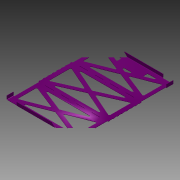
# Autodesk Inventor part: Base
Saved by Autodesk Inventor 2014 (Build 180170000, 170)
## iProperties
Created: 2014-01-11
Part Number: Base
Material: Aluminum 6061
Document SubType Name: Sheet Metal
Designer: Alex
Density: 2.71 g/cm^3
Sheet Metal Rule: Default
Appearance: Smooth - Purple
Mass: 1183.5 g
Surface Area: 4063.5 cm^2
Volume: 436.714 cm^3
Author: Alex
Autodesk Inventor part; units mm, degrees
ref_plane "YZ Plane" through (0, 0, 0) normal (1, 0, 0) x (0, 1, 0)
ref_plane "XZ Plane" through (0, 0, 0) normal (0, 1, 0) x (-1, 0, 0)
ref_plane "XY Plane" through (0, 0, 0) normal (0, 0, 1) x (1, 0, 0)
sketch "Sketch1" plane through (0, 0, 0) normal (0, 1, 0) x (-1, 0, 0)
  line L0 (-666.279, 180.2846) -> (-168.6422, 180.2846)
  line L1 (-168.6422, 180.2846) -> (-168.6422, -512.1194)
  line L2 (-168.6422, -512.1194) -> (-666.279, -512.1194)
  line L3 (-666.279, -512.1194) -> (-666.279, 180.2846)
  line L4 (-666.279, 180.2846) -> (-590.079, 180.2846)
  line L5 (-590.079, 180.2846) -> (-590.079, 175.7126)
  line L6 (-590.079, 175.7126) -> (-666.279, 175.7126)
  line L7 (-666.279, 175.7126) -> (-666.279, 180.2846)
  line L8 (-168.6422, 180.2846) -> (-244.8422, 180.2846)
  line L9 (-244.8422, 180.2846) -> (-244.8422, 175.7126)
  line L10 (-244.8422, 175.7126) -> (-168.6422, 175.7126)
  line L11 (-168.6422, 175.7126) -> (-168.6422, 180.2846)
  line L12 (-666.279, -512.1194) -> (-590.079, -512.1194)
  line L13 (-590.079, -512.1194) -> (-590.079, -507.5474)
  line L14 (-590.079, -507.5474) -> (-666.279, -507.5474)
  line L15 (-666.279, -507.5474) -> (-666.279, -512.1194)
  line L16 (-168.6422, -512.1194) -> (-244.8422, -512.1194)
  line L17 (-244.8422, -512.1194) -> (-244.8422, -507.5474)
  line L18 (-244.8422, -507.5474) -> (-168.6422, -507.5474)
  line L19 (-168.6422, -507.5474) -> (-168.6422, -512.1194)
  line L20 (-666.279, 129.4846) -> (-657.4906, 129.4846)
  line L21 (-657.4906, 129.4846) -> (-657.4906, -461.3194)
  line L22 (-657.4906, -461.3194) -> (-666.279, -461.3194)
  line L23 (-666.279, -461.3194) -> (-666.279, 129.4846)
  line L24 (-168.6422, 129.4846) -> (-177.4306, 129.4846)
  line L25 (-177.4306, 129.4846) -> (-177.4306, -461.3194)
  line L26 (-177.4306, -461.3194) -> (-168.6422, -461.3194)
  line L27 (-168.6422, -461.3194) -> (-168.6422, 129.4846)
  point P0 (0, 0)
  dimension "d0" = 497.6368
  dimension "d1" = 692.404
  dimension "d5" = 76.2
  dimension "d6" = 4.572
  dimension "d7" = 76.2
  dimension "d8" = 4.572
  dimension "d9" = 76.2
  dimension "d10" = 4.572
  dimension "d11" = 76.2
  dimension "d12" = 4.572
  dimension "d13" = 8.7884
  dimension "d15" = 46.228
  dimension "d16" = 46.228
  dimension "d17" = 8.7884
  dimension "d28" = 50.8
  dimension "d29" = 50.8
  dimension "d30" = 50.8
  measures "d0" distance of L1.end L2.end
  measures "d1" distance of L0.end L1.end
  measures "d5" distance of L5.end L6.end
  measures "d6" distance of L4.end L5.end
  measures "d7" distance of L10.end L9.end
  measures "d8" distance of L9.end L8.end
  measures "d9" distance of L14.end L13.end
  measures "d10" distance of L13.end L12.end
  measures "d11" distance of L17.end L18.end
  measures "d12" distance of L16.end L17.end
  measures "d13" distance of L21.end L22.end
  measures "d15" distance between parallel lines of L6 L20
  measures "d16" distance between parallel lines of L14 L22
  measures "d17" distance of L26.end L25.end
  measures "d28" distance between parallel lines of L20 L0
  measures "d29" distance between parallel lines of L0 L24
  measures "d30" distance from line of L25.end L2
extrude "Plate1" add sketch "Sketch1" along normal blind 2.286 contours L0 L9 L10 L1 L24 L25 L26 L18 L17 L2 L13 L14 L3 L22 L21 L20 L6 L5
sketch "Sketch2" plane through (0, 0, 0) normal (0, -1, 0) x (1, 0, 0)
  line L0 (281.5214, -46.0294) -> (281.5214, -43.7434) projected
  line L1 (281.5214, -43.7434) -> (223.2919, -43.7434) projected
  line L2 (223.2919, -43.7434) -> (223.2919, -46.0294) projected
  line L3 (223.2919, -46.0294) -> (281.5214, -46.0294) projected
  line L4 (390.5509, -43.7434) -> (332.3214, -43.7434) projected
  line L5 (390.5509, -46.0294) -> (390.5509, -43.7434) projected
  line L6 (390.5509, -43.7434) -> (332.3214, -43.7434) projected
  line L7 (332.3214, -43.7434) -> (332.3214, -46.0294) projected
  line L8 (332.3214, -46.0294) -> (390.5509, -46.0294) projected
  line L9 (499.5804, -46.0294) -> (499.5804, -43.7434) projected
  line L10 (499.5804, -43.7434) -> (441.3509, -43.7434) projected
  line L11 (441.3509, -43.7434) -> (441.3509, -46.0294) projected
  line L12 (441.3509, -46.0294) -> (499.5804, -46.0294) projected
  line L13 (608.6098, -46.0294) -> (608.6098, -43.7434) projected
  line L14 (608.6098, -43.7434) -> (550.3804, -43.7434) projected
  line L15 (550.3804, -43.7434) -> (550.3804, -46.0294) projected
  line L16 (550.3804, -46.0294) -> (608.6098, -46.0294) projected
  line L17 (223.2919, -288.0914) -> (281.5214, -288.0914) projected
  line L18 (281.5214, -288.0914) -> (281.5214, -285.8054) projected
  line L19 (281.5214, -285.8054) -> (223.2919, -285.8054) projected
  line L20 (223.2919, -285.8054) -> (223.2919, -288.0914) projected
  line L21 (223.2919, -288.0914) -> (281.5214, -288.0914) projected
  line L22 (390.5509, -288.0914) -> (390.5509, -285.8054) projected
  line L23 (390.5509, -285.8054) -> (332.3214, -285.8054) projected
  line L24 (332.3214, -285.8054) -> (332.3214, -288.0914) projected
  line L25 (332.3214, -288.0914) -> (390.5509, -288.0914) projected
  line L26 (441.3509, -288.0914) -> (499.5804, -288.0914) projected
  line L27 (499.5804, -288.0914) -> (499.5804, -285.8054) projected
  line L28 (499.5804, -285.8054) -> (441.3509, -285.8054) projected
  line L29 (441.3509, -285.8054) -> (441.3509, -288.0914) projected
  line L30 (441.3509, -288.0914) -> (499.5804, -288.0914) projected
  line L31 (608.6098, -288.0914) -> (608.6098, -285.8054) projected
  line L32 (608.6098, -285.8054) -> (550.3804, -285.8054) projected
  line L33 (550.3804, -285.8054) -> (550.3804, -288.0914) projected
  line L34 (550.3804, -288.0914) -> (608.6098, -288.0914) projected
  point P0 (0, 0)
extrude "Cut1" cut sketch "Sketch2" against normal blind 2.286
sketch "Sketch3" plane through (244.8422, 0, -509.8334) normal (0, 0, -1) x (-1, 0, 0)
  line L0 (-345.2368, 0) -> (0, 0)
  line L1 (0, 0) -> (0, 25.4)
  line L2 (0, 25.4) -> (-345.2368, 25.4)
  line L3 (-345.2368, 25.4) -> (-345.2368, 0)
  constraints: 6 end point, 1 horizontal, 1 perpendicular, 1 vertical
edge flange "Flange1" height 25.4 angle 90 thickness 2.286 bend radius 2.286 thickness toward (0, 0, -1) relief straight relief width 2.286 relief depth 1.143 corner gap 2.286 corner form 0 edges at (417.4606, 2.286, -512.1194) (168.6422, 2.286, -484.4334) (168.6422, 2.286, 152.5986) (417.4606, 2.286, 180.2846) (666.279, 2.286, 152.5986) (666.279, 2.286, -484.4334) wall of the first edge with corners at (590.079, 0, -509.8334) (244.8422, 0, -509.8334) (244.8422, 25.4, -509.8334) (590.079, 25.4, -509.8334)
bend "Bend1"
corner "Corner1"
sketch "Sketch4" plane through (0, 2.286, 0) normal (0, 1, 0) x (1, 0, 0)
  line L0 (499.5804, 43.7434) -> (441.3509, 43.7434) projected
  line L1 (332.3214, 46.0294) -> (390.5509, 46.0294) projected
  line L2 (390.5509, 285.8054) -> (332.3214, 285.8054) projected
  line L3 (332.3214, 288.0914) -> (390.5509, 288.0914) projected
  line L4 (657.4906, -129.4846) -> (657.4906, 461.3194) projected
  line L5 (590.079, 507.5474) -> (244.8422, 507.5474) projected
  line L6 (177.4306, 461.3194) -> (177.4306, -129.4846) projected
  line L7 (244.8422, -175.7126) -> (590.079, -175.7126) projected
  line L8 (202.8306, 260.4054) -> (632.0906, 260.4054)
  line L9 (632.0906, 260.4054) -> (632.0906, 71.4294)
  line L10 (632.0906, 71.4294) -> (202.8306, 71.4294)
  line L11 (202.8306, 71.4294) -> (202.8306, 260.4054)
  line L12 (632.0906, 313.4914) -> (202.8306, 313.4914)
  line L13 (202.8306, 313.4914) -> (202.8306, 482.1474)
  line L14 (202.8306, 482.1474) -> (632.0906, 482.1474)
  line L15 (632.0906, 482.1474) -> (632.0906, 313.4914)
  line L16 (632.0906, 18.3434) -> (202.8306, 18.3434)
  line L17 (202.8306, 18.3434) -> (202.8306, -150.3126)
  line L18 (202.8306, -150.3126) -> (632.0906, -150.3126)
  line L19 (632.0906, -150.3126) -> (632.0906, 18.3434)
  line L20 (634.079, 312.7101) -> (202.8306, 482.1474)
  line L21 (632.0906, 482.1474) -> (202.8306, 313.4914)
  line L22 (202.8306, 260.4054) -> (632.0906, 71.4294)
  line L23 (632.0906, 260.4054) -> (202.8306, 71.4294)
  line L24 (202.8306, 18.3434) -> (632.0906, -150.3126)
  line L25 (632.0906, 18.3434) -> (202.8306, -150.3126)
  line L26 (632.0906, 327.1365) -> (237.5598, 482.1474)
  line L27 (202.8306, 468.5023) -> (597.3614, 313.4914)
  line L28 (237.5598, 313.4914) -> (632.0906, 468.5023)
  line L29 (202.8306, 327.1365) -> (597.3614, 482.1474)
  line L30 (237.5598, 313.4914) -> (417.4606, 384.1743)
  line L31 (417.4606, 384.1743) -> (597.3614, 313.4914)
  line L32 (597.3614, 313.4914) -> (237.5598, 313.4914)
  line L33 (202.8306, 327.1365) -> (382.7314, 397.8194)
  line L34 (202.8306, 468.5023) -> (202.8306, 327.1365)
  line L35 (382.7314, 397.8194) -> (202.8306, 468.5023)
  line L36 (417.4606, 411.4645) -> (597.3614, 482.1474)
  line L37 (597.3614, 482.1474) -> (237.5598, 482.1474)
  line L38 (237.5598, 482.1474) -> (417.4606, 411.4645)
  line L39 (452.1898, 397.8194) -> (632.0906, 468.5023)
  line L40 (632.0906, 327.1365) -> (632.0906, 468.5023)
  line L41 (632.0906, 327.1365) -> (452.1898, 397.8194)
  line L42 (600.5707, 260.4054) -> (202.8306, 85.3056)
  line L43 (234.3505, 71.4294) -> (632.0906, 246.5292)
  line L44 (202.8306, 246.5292) -> (600.5707, 71.4294)
  line L45 (234.3505, 260.4054) -> (632.0906, 85.3056)
  line L46 (234.3505, 71.4294) -> (417.4606, 152.0412)
  line L47 (417.4606, 152.0412) -> (600.5707, 71.4294)
  line L48 (600.5707, 71.4294) -> (234.3505, 71.4294)
  line L49 (202.8306, 85.3056) -> (385.9407, 165.9174)
  line L50 (385.9407, 165.9174) -> (202.8306, 246.5292)
  line L51 (202.8306, 246.5292) -> (202.8306, 85.3056)
  line L52 (234.3505, 260.4054) -> (600.5707, 260.4054)
  line L53 (600.5707, 260.4054) -> (417.4606, 179.7936)
  line L54 (417.4606, 179.7936) -> (234.3505, 260.4054)
  line L55 (448.9805, 165.9174) -> (632.0906, 246.5292)
  line L56 (448.9805, 165.9174) -> (632.0906, 85.3056)
  line L57 (632.0906, 85.3056) -> (632.0906, 246.5292)
  line L58 (632.0906, -136.6675) -> (237.5598, 18.3434)
  line L59 (202.8306, 4.6983) -> (597.3614, -150.3126)
  line L60 (597.3614, 18.3434) -> (202.8306, -136.6675)
  line L61 (632.0906, 4.6983) -> (237.5598, -150.3126)
  line L62 (237.5598, 18.3434) -> (417.4606, -52.3395)
  line L63 (417.4606, -52.3395) -> (597.3614, 18.3434)
  line L64 (597.3614, 18.3434) -> (223.2919, 18.3434)
  line L65 (382.7314, -65.9846) -> (202.8306, 4.6983)
  line L66 (382.7314, -65.9846) -> (202.8306, -136.6675)
  line L67 (202.8306, -136.6675) -> (202.8306, 4.6983)
  line L68 (237.5598, -150.3126) -> (597.3614, -150.3126)
  line L69 (597.3614, -150.3126) -> (417.4606, -79.6297)
  line L70 (632.0906, 4.6983) -> (632.0906, -136.6675)
  line L71 (632.0906, -136.6675) -> (452.1898, -65.9846)
  line L72 (632.0906, 4.6983) -> (452.1898, -65.9846)
  line L73 (417.4606, -52.3395) -> (597.3614, 18.3434)
  line L74 (597.3614, 18.3434) -> (417.4606, -52.3395)
  line L75 (417.4606, -52.3395) -> (237.5598, 18.3434)
  line L76 (237.5598, 18.3434) -> (597.3614, 18.3434)
  point P0 (657.1239, -129.4846)
  point P1 (657.1239, 461.3194)
  point P2 (177.0639, 461.3194)
  point P3 (177.0639, -129.4846)
  point P4 (0, 0)
  point P5 (177.4306, -129.4846)
  dimension "d31" = 25.4
  dimension "d32" = 25.4
  dimension "d33" = 25.4
  dimension "d34" = 25.4
  dimension "d35" = 25.4
  dimension "d36" = 25.4
  dimension "d37" = 25.4
  dimension "d38" = 25.4
  dimension "d39" = 25.4
  dimension "d40" = 25.4
  dimension "d41" = 25.4
  dimension "d42" = 25.4
  dimension "d43" = 12.7
  dimension "d44" = 12.7
  dimension "d45" = 12.7
  dimension "d47" = 12.7
  dimension "d48" = 12.7
  dimension "d49" = 12.7
  dimension "d50" = 12.7
  dimension "d51" = 12.7
  dimension "d52" = 12.7
  dimension "d53" = 12.7
  dimension "d54" = 12.7
  dimension "d55" = 12.7
  constraints: 138 end point, 51 point on line, 25 parallel, 16 collinear, 8 perpendicular, 3 horizontal, 2 other
  measures "d33" distance between parallel lines of L0 L16
  measures "d34" distance between parallel lines of L18 L7
  measures "d37" distance between parallel lines of L10 L1
  measures "d38" distance between parallel lines of L8 L2
  measures "d39" distance between parallel lines of L12 L3
  measures "d42" distance between parallel lines of L5 L14
  measures "d43" distance between parallel lines of L20 L26
  measures "d44" distance between parallel lines of L20 L27
  measures "d45" distance from line of L12.end L28
  measures "d47" distance from line of L29 L12.end
  measures "d48" distance between parallel lines of L42 L23
  measures "d49" distance between parallel lines of L23 L43
  measures "d50" distance between parallel lines of L22 L44
  measures "d51" distance between parallel lines of L45 L22
  measures "d52" distance between parallel lines of L25 L60
  measures "d53" distance between parallel lines of L25 L61
  measures "d54" distance between parallel lines of L59 L24
  measures "d55" distance between parallel lines of L24 L58
extrude "Cut2" cut sketch "Sketch4" against normal blind 2.286 contours L8 L42 L45 | L44 L42 L11 | L9 L45 L43 | L43 L44 L10 | L12 L28 L27 | L26 L28 L15 | L13 L27 L29 | L29 L26 L14 | L60 L58 L16 | L19 L58 L61 | L60 L17 L59 | L18 L61 L59
fillet "Corner Round1" radius 6.35 12 edges at (417.4606, 1.143, -411.4645) (452.1898, 1.143, -397.8194) (417.4606, 1.143, -384.1743) (382.7314, 1.143, -397.8194) (417.4606, 1.143, -179.7936) (448.9805, 1.143, -165.9174) (417.4606, 1.143, -152.0412) (385.9407, 1.143, -165.9174) (417.4606, 1.143, 79.6297) (417.4606, 1.143, 52.3395) (452.1898, 1.143, 65.9846) (382.7314, 1.143, 65.9846)
fillet "Corner Round2" radius 6.35 24 edges at (202.8306, 1.143, -468.5023) (237.5598, 1.143, -482.1474) (237.5598, 1.143, -313.4914) (202.8306, 1.143, -327.1365) (597.3614, 1.143, -482.1474) (632.0906, 1.143, -468.5023) (632.0906, 1.143, -327.1365) (597.3614, 1.143, -313.4914) (600.5707, 1.143, -260.4054) (632.0906, 1.143, -246.5292) (632.0906, 1.143, -85.3056) (600.5707, 1.143, -71.4294) (234.3505, 1.143, -71.4294) (202.8306, 1.143, -85.3056) (202.8306, 1.143, -246.5292) (234.3505, 1.143, -260.4054) (202.8306, 1.143, -4.6983) (237.5598, 1.143, -18.3434) (597.3614, 1.143, -18.3434) (632.0906, 1.143, -4.6983) (632.0906, 1.143, 136.6675) (597.3614, 1.143, 150.3126) (237.5598, 1.143, 150.3126) (202.8306, 1.143, 136.6675)
sketch "Sketch5" plane through (0, 2.286, 0) normal (0, 1, 0) x (1, 0, 0)
  line L0 (550.3804, 46.0294) -> (608.6098, 46.0294)
  line L1 (657.4906, -129.4846) -> (657.4906, 461.3194)
  line L2 (657.4906, 48.5694) -> (662.0626, 48.5694)
  line L3 (662.0626, 48.5694) -> (662.0626, 283.2654)
  line L4 (662.0626, 283.2654) -> (657.4906, 283.2654)
  line L5 (657.4906, 283.2654) -> (657.4906, 48.5694)
  line L6 (662.0626, 283.2654) -> (664.3486, 283.2654)
  line L7 (664.3486, 283.2654) -> (664.3486, 270.5654)
  line L8 (664.3486, 270.5654) -> (662.0626, 270.5654)
  line L9 (662.0626, 270.5654) -> (662.0626, 283.2654)
  line L10 (662.0626, 93.0194) -> (664.3486, 93.0194)
  line L11 (664.3486, 93.0194) -> (664.3486, 80.3194)
  line L12 (664.3486, 80.3194) -> (662.0626, 80.3194)
  line L13 (662.0626, 80.3194) -> (662.0626, 93.0194)
  line L14 (662.0626, 48.5694) -> (663.9819, 48.5694)
  line L15 (663.9819, 48.5694) -> (663.9819, 61.2694)
  line L16 (663.9819, 61.2694) -> (662.0626, 61.2694)
  line L17 (662.0626, 61.2694) -> (662.0626, 48.5694)
  line L18 (608.6098, 285.8054) -> (550.3804, 285.8054)
  line L19 (662.0626, 112.0694) -> (664.3486, 112.0694)
  line L20 (664.3486, 112.0694) -> (664.3486, 124.7694)
  line L21 (664.3486, 124.7694) -> (662.0626, 124.7694)
  line L22 (662.0626, 124.7694) -> (662.0626, 112.0694)
  line L23 (662.0626, 143.8194) -> (663.9819, 143.8194)
  line L24 (663.9819, 143.8194) -> (663.9819, 156.5194)
  line L25 (663.9819, 156.5194) -> (662.0626, 156.5194)
  line L26 (662.0626, 156.5194) -> (662.0626, 143.8194)
  line L27 (662.0626, 251.5154) -> (663.9819, 251.5154)
  line L28 (663.9819, 251.5154) -> (663.9819, 238.8154)
  line L29 (663.9819, 238.8154) -> (662.0626, 238.8154)
  line L30 (662.0626, 238.8154) -> (662.0626, 251.5154)
  line L31 (662.0626, 219.7654) -> (663.9819, 219.7654)
  line L32 (663.9819, 219.7654) -> (663.9819, 207.0654)
  line L33 (663.9819, 207.0654) -> (662.0626, 207.0654)
  line L34 (662.0626, 207.0654) -> (662.0626, 219.7654)
  line L35 (662.0626, 188.0154) -> (663.9819, 188.0154)
  line L36 (663.9819, 188.0154) -> (663.9819, 185.6248)
  line L37 (662.0626, 185.6248) -> (662.0626, 188.0154)
  line L38 (662.0626, 185.614) -> (662.0626, 165.9174)
  line L39 (664.3486, 185.614) -> (664.3486, 175.5694)
  line L40 (664.3486, 175.5694) -> (662.0626, 175.5694)
  line L41 (662.0626, 175.5694) -> (662.0626, 185.614)
  line L42 (662.0626, 188.0154) -> (664.3486, 188.0154)
  line L43 (664.3486, 188.0154) -> (664.3486, 175.5694)
  line L44 (664.3486, 175.5694) -> (662.0626, 175.5694)
  line L45 (662.0626, 175.5694) -> (662.0626, 188.0154)
  point P0 (657.1239, -129.4846)
  point P1 (657.1239, 461.3194)
  point P2 (0, 0)
  dimension "d60" = 4.572
  dimension "d61" = 2.54
  dimension "d78" = 2.286
  dimension "d79" = 2.286
  dimension "d80" = 12.7
  dimension "d81" = 12.7
  dimension "d82" = 19.05
  dimension "d97" = 2.54
  dimension "d98" = 12.7
  dimension "d99" = 2.286
  dimension "d100" = 19.05
  dimension "d101" = 19.05
  dimension "d102" = 12.7
  dimension "d103" = 12.7
  dimension "d104" = 19.05
  dimension "d105" = 12.7
  dimension "d106" = 19.05
  dimension "d107" = 12.7
  dimension "d108" = 19.05
  dimension "d109" = 19.05
  dimension "d110" = 2.286
  measures "d60" distance of L4.end L4.start
  measures "d61" distance between parallel lines of L2 L0
  measures "d78" distance of L7.end L8.end
  measures "d79" distance of L11.end L12.end
  measures "d80" distance between parallel lines of L16 L14
  measures "d81" distance between parallel lines of L6 L8
  measures "d82" distance between parallel lines of L16 L12
  measures "d97" distance between parallel lines of L18 L4
  measures "d98" distance between parallel lines of L12 L10
  measures "d99" distance of L19.start L19.end
  measures "d100" distance between parallel lines of L10 L19
  measures "d101" distance between parallel lines of L23 L21
  measures "d102" distance between parallel lines of L21 L19
  measures "d103" distance between parallel lines of L23 L25
  measures "d104" distance between parallel lines of L8 L27
  measures "d105" distance between parallel lines of L27 L29
  measures "d106" distance between parallel lines of L29 L31
  measures "d107" distance from line of L31.end L33
  measures "d108" distance between parallel lines of L33 L35
  measures "d109" distance between parallel lines of L40 L25
sheet face with bend "Face2" sketch "Sketch5" thickness 2.286 toward (0, -1, 0) bend radius 2.286 relief straight relief width 2.286 relief depth 1.143
bend "Bend2"
sketch "Sketch7" plane through (0, 2.286, 0) normal (0, 1, 0) x (1, 0, 0)
  line L0 (281.5214, 285.8054) -> (223.2919, 285.8054)
  line L1 (177.4306, 461.3194) -> (177.4306, -129.4846)
  line L2 (177.4306, 283.2654) -> (172.8586, 283.2654)
  line L3 (172.8586, 283.2654) -> (172.8586, 48.5694)
  line L4 (172.8586, 48.5694) -> (177.4306, 48.5694)
  line L5 (177.4306, 48.5694) -> (177.4306, 283.2654)
  line L6 (172.8586, 48.5694) -> (170.5726, 48.5694)
  line L7 (170.5726, 48.5694) -> (170.5726, 61.2694)
  line L8 (170.5726, 61.2694) -> (172.8586, 61.2694)
  line L9 (172.8586, 61.2694) -> (172.8586, 48.5694)
  line L10 (172.8586, 283.2654) -> (170.2059, 283.2654)
  line L11 (170.2059, 283.2654) -> (170.2059, 270.5654)
  line L12 (170.2059, 270.5654) -> (172.8586, 270.5654)
  line L13 (172.8586, 270.5654) -> (172.8586, 283.2654)
  line L14 (172.8586, 80.3194) -> (170.2059, 80.3194)
  line L15 (170.2059, 80.3194) -> (170.2059, 93.0194)
  line L16 (170.2059, 93.0194) -> (172.8586, 93.0194)
  line L17 (172.8586, 93.0194) -> (172.8586, 80.3194)
  line L18 (223.2919, 46.0294) -> (281.5214, 46.0294)
  line L19 (172.8586, 251.5154) -> (170.5726, 251.5154)
  line L20 (170.5726, 251.5154) -> (170.5726, 238.8154)
  line L21 (170.5726, 238.8154) -> (172.8586, 238.8154)
  line L22 (172.8586, 238.8154) -> (172.8586, 251.5154)
  line L23 (172.8586, 112.0694) -> (170.2059, 112.0694)
  line L24 (170.2059, 112.0694) -> (170.2059, 124.7694)
  line L25 (170.2059, 124.7694) -> (172.8586, 124.7694)
  line L26 (172.8586, 124.7694) -> (172.8586, 112.0694)
  line L27 (172.8586, 207.0654) -> (170.5726, 207.0654)
  line L28 (170.5726, 207.0654) -> (170.5726, 219.7654)
  line L29 (170.5726, 219.7654) -> (172.8586, 219.7654)
  line L30 (172.8586, 219.7654) -> (172.8586, 207.0654)
  line L31 (172.8586, 143.8194) -> (170.2059, 143.8194)
  line L32 (170.2059, 143.8194) -> (170.2059, 156.5194)
  line L33 (170.2059, 156.5194) -> (172.8586, 156.5194)
  line L34 (172.8586, 156.5194) -> (172.8586, 143.8194)
  line L35 (172.8586, 172.828) -> (172.8586, 163.1838)
  line L36 (172.8586, 189.2854) -> (170.2059, 189.2854)
  line L37 (170.2059, 189.2854) -> (170.2059, 175.5694)
  line L38 (170.2059, 175.5694) -> (172.8586, 175.5694)
  line L39 (172.8586, 175.5694) -> (172.8586, 189.2854)
  point P0 (177.0639, 461.3194)
  point P1 (177.0639, -129.4846)
  point P2 (0, 0)
  point P3 (177.4306, -129.4846)
  dimension "d84" = 4.572
  dimension "d85" = 2.54
  dimension "d87" = 2.286
  dimension "d88" = 12.7
  dimension "d89" = 12.7
  dimension "d91" = 19.05
  dimension "d112" = 2.54
  dimension "d113" = 12.7
  dimension "d114" = 19.05
  dimension "d115" = 12.7
  dimension "d116" = 19.05
  dimension "d117" = 12.7
  dimension "d118" = 19.05
  dimension "d119" = 2.286
  dimension "d120" = 12.7
  dimension "d121" = 19.05
  dimension "d122" = 12.7
  dimension "d123" = 2.286
  dimension "d124" = 17.78
  dimension "d125" = 19.05
  measures "d84" distance of L4.end L4.start
  measures "d85" distance between parallel lines of L2 L0
  measures "d87" distance of L7.end L8.end
  measures "d88" distance between parallel lines of L6 L8
  measures "d89" distance between parallel lines of L12 L10
  measures "d91" distance between parallel lines of L8 L14
  measures "d112" distance between parallel lines of L18 L4
  measures "d113" distance between parallel lines of L14 L16
  measures "d114" distance between parallel lines of L16 L23
  measures "d115" distance between parallel lines of L23 L25
  measures "d116" distance between parallel lines of L31 L25
  measures "d117" distance between parallel lines of L31 L33
  measures "d118" distance between parallel lines of L19 L12
  measures "d119" distance of L20.end L21.end
  measures "d120" distance from line of L21 L19.start
  measures "d121" distance from line of L29 L21.end
  measures "d122" distance between parallel lines of L29 L27
  measures "d123" distance of L27.start L27.end
  measures "d124" distance between parallel lines of L36 L27
  measures "d125" distance between parallel lines of L33 L38
sheet face with bend "Face3" sketch "Sketch7" thickness 2.286 toward (0, -1, 0) bend radius 2.286 relief straight relief width 2.286 relief depth 1.143
bend "Bend4"
sketch "Sketch8" plane through (590.079, 25.4, 177.9986) normal (0, 0, -1) x (-1, 0, 0)
  circle A0 centre (432.573, 25.4) radius 1.5875 projected
  circle A1 centre (-86.603, 25.4) radius 1.5875 projected
  circle A2 centre (51.5333, -12.7) radius 1.5875 projected
  circle A3 centre (295.1701, -12.7) radius 1.5875 projected
  line L0 (514.107, 128.016) -> (514.107, 129.286) projected
  line L1 (514.107, 129.286) -> (271.41, 129.286) projected
  line L2 (-168.137, 129.286) -> (-168.137, 128.016) projected
  line L3 (-168.137, 128.016) -> (-170.677, 128.016) projected
  line L4 (-170.677, 128.016) -> (-170.677, 127) projected
  line L5 (-170.677, 127) -> (-173.217, 127) projected
  line L6 (-173.217, 101.6) -> (-173.217, 127) projected
  line L7 (-173.217, 101.6) -> (-170.677, 101.6) projected
  line L8 (-170.677, 101.6) -> (-170.677, 76.2) projected
  line L9 (-170.677, 76.2) -> (-173.217, 76.2) projected
  line L10 (-173.217, 25.4) -> (-173.217, 76.2) projected
  line L11 (-173.217, 25.4) -> (-170.677, 25.4) projected
  line L12 (-170.677, 25.4) -> (-170.677, 0) projected
  line L13 (-170.677, 0) -> (-173.217, 0) projected
  line L14 (-173.217, -25.4) -> (-173.217, 0) projected
  line L15 (-173.217, -25.4) -> (519.187, -25.4) projected
  line L16 (519.187, 0) -> (519.187, -25.4) projected
  line L17 (519.187, 0) -> (516.647, 0) projected
  line L18 (516.647, 0) -> (516.647, 25.4) projected
  line L19 (516.647, 25.4) -> (519.187, 25.4) projected
  line L20 (519.187, 76.2) -> (519.187, 25.4) projected
  line L21 (519.187, 76.2) -> (516.647, 76.2) projected
  line L22 (516.647, 76.2) -> (516.647, 101.6) projected
  line L23 (516.647, 101.6) -> (519.187, 101.6) projected
  line L24 (519.187, 127) -> (519.187, 101.6) projected
  line L25 (519.187, 127) -> (516.647, 127) projected
  line L26 (516.647, 127) -> (516.647, 128.016) projected
  line L27 (516.647, 128.016) -> (514.107, 128.016) projected
  line L28 (-135.6043, 64.3588) -> (-109.8383, 2.4396) projected
  arc A4 (-115.701, -6.35) -> (-109.8383, 2.4396) centre (-115.701, 0) ccw projected
  line L29 (-115.701, -6.35) -> (-141.467, -6.35) projected
  arc A5 (-147.817, 0) -> (-141.467, -6.35) centre (-141.467, 0) ccw projected
  line L30 (-147.817, 0) -> (-147.817, 61.9192) projected
  arc A6 (-135.6043, 64.3588) -> (-147.817, 61.9192) centre (-141.467, 61.9192) ccw projected
  line L31 (455.8084, 2.4396) -> (481.5744, 64.3588) projected
  arc A7 (493.787, 61.9192) -> (481.5744, 64.3588) centre (487.437, 61.9192) ccw projected
  line L32 (493.787, 61.9192) -> (493.787, 0) projected
  arc A8 (487.437, -6.35) -> (493.787, 0) centre (487.437, 0) ccw projected
  line L33 (487.437, -6.35) -> (461.6711, -6.35) projected
  arc A9 (455.8084, 2.4396) -> (461.6711, -6.35) centre (461.6711, 0) ccw projected
  line L34 (483.2517, 101.4464) -> (457.4857, 39.5272) projected
  arc A10 (445.273, 41.9668) -> (457.4857, 39.5272) centre (451.623, 41.9668) ccw projected
  line L35 (445.273, 41.9668) -> (445.273, 103.886) projected
  arc A11 (451.623, 110.236) -> (445.273, 103.886) centre (451.623, 103.886) ccw projected
  line L36 (451.623, 110.236) -> (477.389, 110.236) projected
  arc A12 (483.2517, 101.4464) -> (477.389, 110.236) centre (477.389, 103.886) ccw projected
  line L37 (-111.5156, 39.5272) -> (-137.2816, 101.4464) projected
  arc A13 (-131.4189, 110.236) -> (-137.2816, 101.4464) centre (-131.4189, 103.886) ccw projected
  line L38 (-131.4189, 110.236) -> (-105.653, 110.236) projected
  arc A14 (-99.303, 103.886) -> (-105.653, 110.236) centre (-105.653, 103.886) ccw projected
  line L39 (-99.303, 103.886) -> (-99.303, 41.9668) projected
  arc A15 (-111.5156, 39.5272) -> (-99.303, 41.9668) centre (-105.653, 41.9668) ccw projected
  arc A16 (287.92, 78.4749) -> (281.57, 78.4749) centre (284.745, 85.402) ccw projected
  line L40 (287.92, 78.4749) -> (287.92, 72.702) projected
  arc A17 (281.57, 72.702) -> (287.92, 72.702) centre (284.745, 72.702) ccw projected
  line L41 (281.57, 72.702) -> (281.57, 78.4749) projected
  arc A18 (64.4, 78.4749) -> (58.05, 78.4749) centre (61.225, 85.402) ccw projected
  line L42 (64.4, 78.4749) -> (64.4, 72.702) projected
  arc A19 (58.05, 72.702) -> (64.4, 72.702) centre (61.225, 72.702) ccw projected
  line L43 (58.05, 72.702) -> (58.05, 78.4749) projected
  arc A20 (-53.71, 72.702) -> (-47.36, 72.702) centre (-50.535, 72.702) ccw projected
  line L44 (-53.71, 72.702) -> (-53.71, 78.4749) projected
  arc A21 (-47.36, 78.4749) -> (-53.71, 78.4749) centre (-50.535, 85.402) ccw projected
  line L45 (-47.36, 78.4749) -> (-47.36, 72.702) projected
  arc A22 (399.68, 78.4749) -> (393.33, 78.4749) centre (396.505, 85.402) ccw projected
  line L46 (399.68, 78.4749) -> (399.68, 72.702) projected
  arc A23 (393.33, 72.702) -> (399.68, 72.702) centre (396.505, 72.702) ccw projected
  line L47 (393.33, 72.702) -> (393.33, 78.4749) projected
  line L48 (227.6601, 97.564) -> (222.9489, 100.046) projected
  arc A24 (225.9087, 112.014) -> (222.9489, 100.046) centre (225.9087, 105.664) ccw projected
  line L49 (225.9087, 112.014) -> (351.9634, 112.014) projected
  arc A25 (354.9232, 100.046) -> (351.9634, 112.014) centre (351.9634, 105.664) ccw projected
  line L50 (354.9232, 100.046) -> (350.212, 97.564) projected
  arc A26 (347.2522, 96.832) -> (350.212, 97.564) centre (347.2522, 103.182) ccw projected
  line L51 (347.2522, 96.832) -> (230.6199, 96.832) projected
  arc A27 (227.6601, 97.564) -> (230.6199, 96.832) centre (230.6199, 103.182) ccw projected
  line L52 (-4.2419, 97.564) -> (-8.9531, 100.046) projected
  arc A28 (-5.9933, 112.014) -> (-8.9531, 100.046) centre (-5.9933, 105.664) ccw projected
  line L53 (-5.9933, 112.014) -> (120.0614, 112.014) projected
  arc A29 (123.0212, 100.046) -> (120.0614, 112.014) centre (120.0614, 105.664) ccw projected
  line L54 (123.0212, 100.046) -> (118.31, 97.564) projected
  arc A30 (115.3502, 96.832) -> (118.31, 97.564) centre (115.3502, 103.182) ccw projected
  line L55 (115.3502, 96.832) -> (-1.2821, 96.832) projected
  arc A31 (-4.2419, 97.564) -> (-1.2821, 96.832) centre (-1.2821, 103.182) ccw projected
  line L56 (-52.567, 66.109) -> (-0.6008, 66.109) projected
  arc A32 (2.359, 65.377) -> (-0.6008, 66.109) centre (-0.6008, 59.759) ccw projected
  line L57 (2.359, 65.377) -> (19.1233, 56.545) projected
  arc A33 (19.1233, 45.309) -> (19.1233, 56.545) centre (16.1635, 50.927) ccw projected
  line L58 (19.1233, 45.309) -> (-49.6072, 9.0994) projected
  arc A34 (-58.917, 14.7174) -> (-49.6072, 9.0994) centre (-52.567, 14.7174) ccw projected
  line L59 (-58.917, 14.7174) -> (-58.917, 59.759) projected
  arc A35 (-52.567, 66.109) -> (-58.917, 59.759) centre (-52.567, 59.759) ccw projected
  line L60 (346.5709, 66.109) -> (398.537, 66.109) projected
  line L61 (175.9448, 96.1) -> (251.0253, 56.545) projected
  arc A36 (251.0253, 45.309) -> (251.0253, 56.545) centre (248.0655, 50.927) ccw projected
  line L62 (251.0253, 45.309) -> (175.9448, 5.754) projected
  arc A37 (170.0253, 5.754) -> (175.9448, 5.754) centre (172.985, 11.372) ccw projected
  line L63 (170.0253, 5.754) -> (94.9448, 45.309) projected
  arc A38 (94.9448, 56.545) -> (94.9448, 45.309) centre (97.9046, 50.927) ccw projected
  line L64 (94.9448, 56.545) -> (170.0253, 96.1) projected
  line L65 (100.2943, 0.254) -> (13.7738, 0.254) projected
  arc A39 (10.814, 12.222) -> (13.7738, 0.254) centre (13.7738, 6.604) ccw projected
  line L66 (10.814, 12.222) -> (54.0743, 35.013) projected
  arc A40 (59.9938, 35.013) -> (54.0743, 35.013) centre (57.034, 29.395) ccw projected
  line L67 (59.9938, 35.013) -> (103.254, 12.222) projected
  arc A41 (100.2943, 0.254) -> (103.254, 12.222) centre (100.2943, 6.604) ccw projected
  line L68 (332.1963, 0.254) -> (245.6758, 0.254) projected
  arc A42 (242.716, 12.222) -> (245.6758, 0.254) centre (245.6758, 6.604) ccw projected
  line L69 (242.716, 12.222) -> (285.9763, 35.013) projected
  arc A43 (291.8958, 35.013) -> (285.9763, 35.013) centre (288.936, 29.395) ccw projected
  line L70 (291.8958, 35.013) -> (335.156, 12.222) projected
  arc A44 (332.1963, 0.254) -> (335.156, 12.222) centre (332.1963, 6.604) ccw projected
  arc A45 (404.887, 59.759) -> (398.537, 66.109) centre (398.537, 59.759) ccw projected
  line L71 (404.887, 59.759) -> (404.887, 14.7174) projected
  arc A46 (395.5773, 9.0994) -> (404.887, 14.7174) centre (398.537, 14.7174) ccw projected
  line L72 (395.5773, 9.0994) -> (326.8468, 45.309) projected
  arc A47 (326.8468, 56.545) -> (326.8468, 45.309) centre (329.8066, 50.927) ccw projected
  line L73 (326.8468, 56.545) -> (343.6111, 65.377) projected
  arc A48 (346.5709, 66.109) -> (343.6111, 65.377) centre (346.5709, 59.759) ccw projected
  circle A49 centre (51.5333, -12.7) radius 1.5875 projected
  circle A50 centre (295.1701, -12.7) radius 1.5875 projected
  line L74 (271.41, 129.286) -> (74.56, 129.286) projected
  line L75 (74.56, 129.286) -> (-168.137, 129.286) projected
  arc A51 (175.9448, 96.1) -> (170.0253, 96.1) centre (172.985, 90.482) ccw projected
  circle A52 centre (293, 51.0485) radius 1.5875 projected
  circle A53 centre (52.97, 51.0485) radius 1.5875 projected
  point P0 (590.079, -25.4)
extrude "Cut3" cut sketch "Sketch8" along normal through all contours A2 | A3
sketch "Sketch9" plane through (0, 2.286, 0) normal (0, 1, 0) x (1, 0, 0)
  line L0 (509.1689, 433.6334) -> (325.0189, 433.6334)
  line L1 (509.1689, 509.8334) -> (509.1689, 433.6334)
  line L2 (325.0189, 509.8334) -> (509.1689, 509.8334)
  line L3 (325.0189, 433.6334) -> (325.0189, 509.8334)
  point P0 (0, 0)
sheet face with bend "Face4" sketch "Sketch9" thickness 2.286 toward (0, -1, 0) bend radius 2.286 relief straight relief width 2.286 relief depth 1.143
bend "Bend5"
fillet "Corner Round3" radius 6.35 6 edges at (325.0189, 1.143, -482.1474) (325.0189, 1.143, -447.7848) (361.0367, 1.143, -433.6334) (473.8845, 1.143, -433.6334) (509.1689, 1.143, -447.4967) (509.1689, 1.143, -482.1474)
sketch "Sketch10" plane through (244.8422, 25.4, 180.2846) normal (0, 0, 1) x (1, 0, 0)
  circle A0 centre (50.8, -12.7) radius 1.5875 projected
  circle A1 centre (294.4368, -12.7) radius 1.5875 projected
  point P0 (-244.8422, -25.4)
extrude "Cut4" cut sketch "Sketch10" against normal through all
sketch "Sketch11" plane through (0, 2.286, 0) normal (0, 1, 0) x (1, 0, 0)
  line L0 (441.3509, 288.0914) -> (499.5804, 288.0914) projected
  line L1 (499.5804, 43.7434) -> (441.3509, 43.7434) projected
  line L2 (332.3214, 46.0294) -> (390.5509, 46.0294) projected
  line L3 (390.5509, 285.8054) -> (332.3214, 285.8054) projected
  circle A0 centre (417.4606, 272.8514) radius 1.5875
  circle A1 centre (417.4606, 301.0454) radius 1.5875
  circle A2 centre (417.4606, 58.9834) radius 1.5875
  circle A3 centre (417.4606, 30.7894) radius 1.5875
  point P0 (0, 0)
  dimension "d136" = 3.175
  dimension "d137" = 12.954
  dimension "d138" = 12.954
  dimension "d139" = 3.175
  dimension "d140" = 3.175
  dimension "d141" = 12.954
  dimension "d142" = 12.954
  constraints: 4 centre point
  measures "d136" diameter of A0
  measures "d137" distance from line of L3 A0.centre
  measures "d138" distance from line of L0 A1.centre
  measures "d139" diameter of A2
  measures "d140" diameter of A3
  measures "d141" distance from line of L1 A3.centre
  measures "d142" distance from line of L2 A2.centre
extrude "Cut5" cut sketch "Sketch11" against normal blind 2.286
equation "\"d15\" = d16"
equation "\"d3\" = Thickness"
equation "\"d56\" = Thickness"
equation "\"d18\" = BendReliefWidth"
equation "\"d19\" = BendReliefDepth"
equation "\"d20\" = MinimumRemnant"
equation "\"d21\" = BendRadius"
equation "\"d24\" = BendRadius"
equation "\"d25\" = CornerReliefSize"
equation "\"d26\" = GapSize"
equation "\"d27\" = JacobiRadiusSize"
equation "\"d63\" = BendRadius"
equation "\"d64\" = BendReliefWidth"
equation "\"d66\" = MinimumRemnant"
equation "\"d65\" = BendReliefDepth"
equation "\"d67\" = BendRadius"
equation "\"d92\" = BendRadius"
equation "\"d93\" = BendReliefWidth"
equation "\"d95\" = MinimumRemnant"
equation "\"d94\" = BendReliefDepth"
equation "\"d96\" = BendRadius"
equation "\"BendRadius\" = Thickness"
equation "\"BendReliefWidth\" = Thickness"
equation "\"BendReliefDepth\" = 0.5 * Thickness"
equation "\"CornerReliefSize\" = 4 * Thickness"
equation "\"MinimumRemnant\" = 2 * Thickness"
equation "\"TransitionRadius\" = BendRadius"
equation "\"JacobiRadiusSize\" = BendRadius"
equation "\"GapSize\" = Thickness"
equation "\"d2\" = BendRadius"
equation "\"Thickness\" = 2.286"
body "Solid1"
